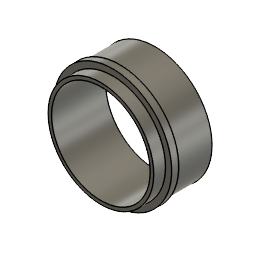
Fan adapter (Autodesk Fusion 360 design; units mm, degrees)
Autodesk Fusion 360 part; units mm, degrees
sketch "Sketch1" plane through (0, 0, 0) normal (0, 0, 1) x (1, 0, 0)
  circle A0 centre (0, 0) radius 25
  dimension "d1" = 50
  constraint coincident A0.centre origin
  measures "d1" diameter of A0
extrude "Extrude1" add sketch "Sketch1" along normal blind 3 makes body 1
sketch "Sketch2" plane through (0, 0, 0) normal (0, 0, -1) x (-1, 0, 0)
  circle A0 centre (0, 0) radius 25
  circle A1 centre (0, 0) radius 22.4
  circle A2 centre (0, 0) radius 20.9
  dimension "d4" = 44.8
  dimension "d5" = -1.5
  constraint coincident A0.centre A1.centre
  measures "d4" diameter of A1
extrude "Extrude2" cut sketch "Sketch2" against normal blind 3 contours A2 bodies 1
extrude "Extrude3" add sketch "Sketch2" against normal blind 8 contours A1 bodies 1
copy_body "Body->Comp1" bodies 1 removing the originals makes body 2 in component "Component"
sketch "Sketch3" plane through (0, 0, 8) normal (0, 0, 1) x (1, 0, 0)
  circle A0 centre (0, 0) radius 20.9
  circle A1 centre (0, 0) radius 22.4
  circle A2 centre (0, 0) radius 22.65
  line L0 (30, -30) -> (-30, -30)
  line L1 (-30, -30) -> (-30, 30)
  line L2 (-30, 30) -> (30, 30)
  line L3 (30, 30) -> (30, -30)
  line L4 (30, -30) -> (-30, 30) construction
  line L5 (-30, -30) -> (30, 30) construction
  dimension "d10" = 0.25
  dimension "d11" = 60
  dimension "d12" = 60
  constraint horizontal L0
  constraint perpendicular L0 L1
  constraint parallel L0 L2
  constraint parallel L1 L3
  constraint coincident L4 A0.centre
  constraint coincident L5 A0.centre
  constraint coincident A0.centre A1.centre
  measures "d11" distance of L1.end L2.end
  measures "d12" distance of L0.end L1.end
extrude "Extrude4" add sketch "Sketch3" against normal blind 5 separate body contours L0 L1 L2 L3 makes body 3
sketch "Sketch4" plane through (0, 0, 8) normal (0, 0, 1) x (1, 0, 0)
  circle A0 centre (0, 0) radius 22.65
  line L0 (30, 30) -> (-30, 30)
  line L1 (-30, 30) -> (-30, -30)
  line L2 (-30, -30) -> (30, -30)
  line L3 (30, -30) -> (30, 30)
  line L4 (-5, -25) -> (5, -25)
  line L5 (5, -25) -> (5, -30)
  line L6 (5, -30) -> (-5, -30)
  line L7 (-5, -30) -> (-5, -25)
  circle A1 centre (-25.5, 25.5) radius 2.5
  circle A2 centre (-25.5, -25.5) radius 2.5
  circle A3 centre (25.5, -25.5) radius 2.5
  circle A4 centre (25.5, 25.5) radius 2.5
  circle A5 centre (-25.5, 25.5) radius 3.5
  circle A6 centre (-25.5, -25.5) radius 3.5
  circle A7 centre (25.5, -25.5) radius 3.5
  circle A8 centre (25.5, 25.5) radius 3.5
  dimension "d15" = 5
  dimension "d16" = 4.5
  dimension "d17" = 4.5
  dimension "d19" = 360
  dimension "d22" = 5
  dimension "d23" = 1
  dimension "d27" = 360
  constraint horizontal L4
  constraint vertical L5
  constraint horizontal L6
  constraint vertical L7
  constraint coincident L2 L5.end
  measures "d15" diameter of A1
  measures "d16" distance of L1 A1.centre
  measures "d17" distance of L0 A1.centre
  measures "d22" distance of L4 L6
extrude "Extrude5" cut sketch "Sketch4" against normal blind 5 contours L2 L4 L5 L6 L7 | A1 | A2 | A3 | A4 bodies 3
extrude "Extrude7" cut sketch "Sketch4" against normal blind 2 contours A5 | A6 | A7 | A8 bodies 3
sketch "Sketch5" plane through (0, 0, 8) normal (0, 0, 1) x (1, 0, 0)
  circle A0 centre (25.5, 25.5) radius 3.5
  circle A1 centre (25.5, -25.5) radius 3.5
  circle A2 centre (-25.5, 25.5) radius 3.5
  circle A3 centre (-25.5, -25.5) radius 3.5
  line L0 (5, -25) -> (5, -30)
  line L1 (5, -30) -> (30, -30)
  line L2 (30, -30) -> (30, 30)
  line L3 (30, 30) -> (-30, 30)
  line L4 (-30, 30) -> (-30, -30)
  line L5 (-30, -30) -> (-5, -30)
  line L6 (-5, -30) -> (-5, -25)
  line L7 (-5, -25) -> (5, -25)
  circle A4 centre (0, 0) radius 22.65
  circle A5 centre (-26.5, 0) radius 2.5
  circle A6 centre (26.5, 0) radius 2.5
  circle A7 centre (0, 26.5) radius 2.5
  point P0 (-22.65, 0)
  dimension "d30" = 5
  dimension "d31" = 3.5
  dimension "d33" = 360
  constraint collinear A5.centre A4.centre P0
  measures "d30" diameter of A5
  measures "d31" distance of L4 A5.centre
extrude "Extrude8" cut sketch "Sketch5" against normal blind 5 contours A5 | A6 | A7 bodies 3
sketch "Sketch6" plane through (0, 0, 3) normal (0, 0, -1) x (-1, 0, 0)
  circle A0 centre (26.5, 0) radius 2.5
  circle A1 centre (0, 26.5) radius 2.5
  circle A2 centre (-26.5, 0) radius 2.5
  line L0 (-5, -30) -> (-5, -25)
  line L1 (-5, -25) -> (5, -25)
  line L2 (5, -25) -> (5, -30)
  line L3 (5, -30) -> (30, -30)
  line L4 (30, -30) -> (30, 30)
  line L5 (30, 30) -> (-30, 30)
  line L6 (-30, 30) -> (-30, -30)
  line L7 (-30, -30) -> (-5, -30)
  circle A3 centre (0, 0) radius 22.65
  circle A4 centre (25.5, 25.5) radius 2.5
  circle A5 centre (25.5, -25.5) radius 2.5
  circle A6 centre (-25.5, 25.5) radius 2.5
  circle A7 centre (-25.5, -25.5) radius 2.5
  circle A8 centre (0, 26.5) radius 3
  circle A9 centre (-26.5, 0) radius 3
  circle A10 centre (26.5, 0) radius 3
  dimension "d36" = 0.5
  dimension "d38" = 360
extrude "Extrude9" cut sketch "Sketch6" against normal blind 2 contours A8 | A9 | A10 bodies 3
copy_body "Body->Comp2" bodies 3 removing the originals makes body 4 in component "Component'"
sketch "Sketch7" plane through (0, 0, 0) normal (0, 0, -1) x (-1, 0, 0)
  circle A0 centre (0, 0) radius 20.9
  circle A1 centre (0, 0) radius 25
  circle A2 centre (0, 0) radius 24.15
  dimension "d41" = 48.3
  constraint coincident A0.centre A1.centre
  measures "d41" diameter of A2
extrude "Extrude1'" add sketch "Sketch7" along normal blind 15 contours A2 bodies 2 in component "Component"
component "Component" placed x (1, 0, 0) y (0, 1, 0) z (0, 0, 1) at (0, 0, 0)
component "Component'" placed x (1, 0, 0) y (0, 1, 0) z (0, 0, 1) at (0, 0, 0)
